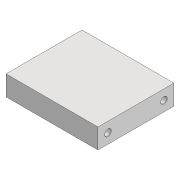
# Autodesk Inventor part: Стенкка для ковнейера
Saved by Autodesk Inventor 2022 (Build 260153000, 153)
## iProperties
Created: 2023-02-18
Part Number: Стенкка для ковнейера
Material: Типовые
Document SubType Name: Modeling
Designer: Глеб
Density: 1 g/cm^3
Appearance: По умолчанию
Author: Глеб
Autodesk Inventor part; units mm, degrees
ref_plane "YZ Plane" through (0, 0, 0) normal (1, 0, 0) x (0, 1, 0)
ref_plane "XZ Plane" through (0, 0, 0) normal (0, 1, 0) x (-1, 0, 0)
ref_plane "XY Plane" through (0, 0, 0) normal (0, 0, 1) x (1, 0, 0)
sketch "Эскиз1" plane through (0, 0, 0) normal (1, 0, 0) x (0, 1, 0)
  line L0 (0, 19) -> (10, 19)
  line L1 (10, 19) -> (10, -19)
  line L2 (10, -19) -> (0, -19)
  line L3 (0, -19) -> (0, 19)
  line L4 (-2, 0) -> (12, 0) construction
  line L5 (0, -26.6) -> (0, 26.6) construction
  point P0 (0, 0)
  dimension "d0" = 10
  dimension "d1" = 38
  constraints: 8 end point, 2 parallel, 1 horizontal, 1 perpendicular, 1 other
  measures "d0" distance of L1.end L2.end
  measures "d1" distance of L0.end L1.end
extrude "Выдавливание1" add sketch "Эскиз1" along normal blind 46
sketch "Эскиз2" plane through (46, 0, 0) normal (1, 0, 0) x (0, 0, -1)
  line L0 (19, 10) -> (-19, 10) projected
  line L1 (-19, 10) -> (-19, 0) projected
  line L2 (19, 0) -> (19, 10) projected
  line L3 (0, -2) -> (0, 12) construction
  point P0 (0, 0)
  point P1 (-14, 5)
  point P2 (14, 5)
  dimension "d4" = 5
  dimension "d5" = 5
  dimension "d6" = 5
  measures "d4" distance from line of L0 point (-14, 5)
  measures "d5" distance from line of L1 point (-14, 5)
  measures "d6" distance from line of point (14, 5) L2
hole "Отверстие1" at (46, 5, 14) at (46, 5, -14) direction (-1, 0, 0) diameter 3 depth 60
chamfer "Фаска1" distance 0.2 angle 45 4 edges at (46, 5, -12.5) (46, 5, 15.5) (0, 5, -12.5) (0, 5, 15.5)
equation "\"d6\" = d5"
